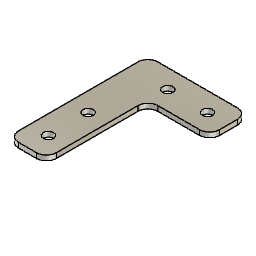
Master v16 (Autodesk Fusion 360 archive; units mm, degrees)
design "Funky Bracket"
Autodesk Fusion 360 part; units mm, degrees
note: some values were not read from the file. Chosen so that the rebuilt part matches the saved one: which face or edge a step refers to. Set by a fixed rule: which sketch regions a step uses.
sketch "Sketch1" plane through (0, 0, 0) normal (0, 0, 1) x (1, 0, 0)
  circle A0 centre (0, -38.1) radius 3.2385
  circle A1 centre (0, -63.5) radius 3.2385
  circle A2 centre (12.7, 0) radius 3.2385
  circle A3 centre (38.1, 0) radius 3.2385
  line L0 (-12.065, 12.065) -> (-12.065, -76.835)
  line L1 (-12.065, -76.835) -> (12.065, -76.835)
  line L2 (12.065, -76.835) -> (12.065, -12.065)
  line L3 (12.065, -12.065) -> (51.435, -12.065)
  line L4 (51.435, -12.065) -> (51.435, 12.065)
  line L5 (51.435, 12.065) -> (-12.065, 12.065)
  line L6 (0, 0) -> (51.435, 0) construction
  line L7 (0, 0) -> (0, -76.835) construction
  dimension "d1" = 6.477
  dimension "d2" = 38.1
  dimension "d4" = 25.4
  dimension "d6" = 12.7
  dimension "d8" = 24.13
  dimension "d9" = 24.13
  dimension "d10" = 88.9
  dimension "d11" = 25.4
  dimension "d12" = 63.5
  constraint equal A0 A1
  constraint equal A0 A2
  constraint equal A2 A3
  constraint vertical L0
  constraint perpendicular L0 L1
  constraint perpendicular L1 L2
  constraint perpendicular L0 L3
  constraint perpendicular L3 L4
  constraint horizontal L5
  constraint coincident L6.start L7.start
  constraint midpoint L4 L6.end
  constraint midpoint L1 L7.end
  constraint vertical L7
  constraint horizontal L6
  measures "d1" diameter of A0
  measures "d2" distance of L6.start A0.centre
  measures "d4" distance of A0.centre A1.centre
  measures "d6" distance of L6.start A2.centre
  measures "d8" distance of L3.end L4.end
  measures "d9" distance of L0.end L1.end
  measures "d10" distance of L0.start L0.end
  measures "d11" distance of A2.centre A3.centre
  measures "d12" distance of L0.start L4.end
extrude "Extrude1" add sketch "Sketch1" along normal blind 3.175
fillet "Fillet1" radius 6.35 6 edges at (12.065, -76.835, 1.5875) (-12.065, -76.835, 1.5875) (-12.065, 12.065, 1.5875) (51.435, -12.065, 1.5875) (51.435, 12.065, 1.5875) (12.065, -12.065, 1.5875)
equation "d13 = ( 1 / 8 ) * 1 in"

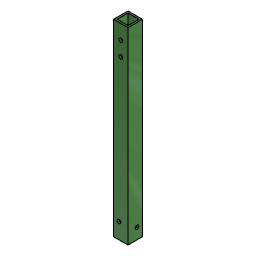
design "Verticle Tube Rear Left"
Autodesk Fusion 360 part; units mm, degrees
imported_body "Derived Base Feature4" makes body 1
imported_body "Derived Base Feature3" makes body 2
sketch "sketch 209" plane through (0, 0, 0) normal (0, 0, 1) x (-1, 0, 0)
  line L0 (-100.8889, 72.7861) -> (-103.3889, 70.7861)
  arc A0 (-109.0111, 77.8139) -> (-103.3889, 70.7861) centre (-106.2, 74.3) ccw
  line L1 (-109.0111, 77.8139) -> (-106.5111, 79.8139)
  arc A1 (-100.8889, 72.7861) -> (-106.5111, 79.8139) centre (-103.7, 76.3) ccw
  line L2 (-106.5111, 821.8861) -> (-109.0111, 823.8861)
  arc A2 (-103.3889, 830.9139) -> (-109.0111, 823.8861) centre (-106.2, 827.4) ccw
  line L3 (-103.3889, 830.9139) -> (-100.8889, 828.9139)
  arc A3 (-106.5111, 821.8861) -> (-100.8889, 828.9139) centre (-103.7, 825.4) ccw
  line L4 (-665.3111, 821.8861) -> (-667.8111, 823.8861)
  arc A4 (-662.1889, 830.9139) -> (-667.8111, 823.8861) centre (-665, 827.4) ccw
  line L5 (-662.1889, 830.9139) -> (-659.6889, 828.9139)
  arc A5 (-665.3111, 821.8861) -> (-659.6889, 828.9139) centre (-662.5, 825.4) ccw
  line L6 (-604.6889, 79.8139) -> (-602.1889, 77.8139)
  arc A6 (-607.8111, 70.7861) -> (-602.1889, 77.8139) centre (-605, 74.3) ccw
  line L7 (-607.8111, 70.7861) -> (-610.3111, 72.7861)
  arc A7 (-604.6889, 79.8139) -> (-610.3111, 72.7861) centre (-607.5, 76.3) ccw
  line L8 (-659.6889, 72.7861) -> (-662.1889, 70.7861)
  arc A8 (-667.8111, 77.8139) -> (-662.1889, 70.7861) centre (-665, 74.3) ccw
  line L9 (-667.8111, 77.8139) -> (-665.3111, 79.8139)
  arc A9 (-659.6889, 72.7861) -> (-665.3111, 79.8139) centre (-662.5, 76.3) ccw
  line L10 (-604.6889, 752.9139) -> (-602.1889, 750.9139)
  arc A10 (-607.8111, 743.8861) -> (-602.1889, 750.9139) centre (-605, 747.4) ccw
  line L11 (-607.8111, 743.8861) -> (-610.3111, 745.8861)
  arc A11 (-604.6889, 752.9139) -> (-610.3111, 745.8861) centre (-607.5, 749.4) ccw
  line L12 (-100.8889, 745.8861) -> (-103.3889, 743.8861)
  arc A12 (-109.0111, 750.9139) -> (-103.3889, 743.8861) centre (-106.2, 747.4) ccw
  line L13 (-109.0111, 750.9139) -> (-106.5111, 752.9139)
  arc A13 (-100.8889, 745.8861) -> (-106.5111, 752.9139) centre (-103.7, 749.4) ccw
  line L14 (-45.8889, 79.8139) -> (-43.3889, 77.8139)
  arc A14 (-49.0111, 70.7861) -> (-43.3889, 77.8139) centre (-46.2, 74.3) ccw
  line L15 (-49.0111, 70.7861) -> (-51.5111, 72.7861)
  arc A15 (-45.8889, 79.8139) -> (-51.5111, 72.7861) centre (-48.7, 76.3) ccw
  line L16 (-106.5111, 148.7861) -> (-109.0111, 150.7861)
  arc A16 (-103.3889, 157.8139) -> (-109.0111, 150.7861) centre (-106.2, 154.3) ccw
  line L17 (-103.3889, 157.8139) -> (-100.8889, 155.8139)
  arc A17 (-106.5111, 148.7861) -> (-100.8889, 155.8139) centre (-103.7, 152.3) ccw
  line L18 (-43.3889, 823.8861) -> (-45.8889, 821.8861)
  arc A18 (-51.5111, 828.9139) -> (-45.8889, 821.8861) centre (-48.7, 825.4) ccw
  line L19 (-51.5111, 828.9139) -> (-49.0111, 830.9139)
  arc A19 (-43.3889, 823.8861) -> (-49.0111, 830.9139) centre (-46.2, 827.4) ccw
  line L20 (-602.1889, 823.8861) -> (-604.6889, 821.8861)
  arc A20 (-610.3111, 828.9139) -> (-604.6889, 821.8861) centre (-607.5, 825.4) ccw
  line L21 (-610.3111, 828.9139) -> (-607.8111, 830.9139)
  arc A21 (-602.1889, 823.8861) -> (-607.8111, 830.9139) centre (-605, 827.4) ccw
  line L22 (-602.1889, 150.7861) -> (-604.6889, 148.7861)
  arc A22 (-610.3111, 155.8139) -> (-604.6889, 148.7861) centre (-607.5, 152.3) ccw
  line L23 (-610.3111, 155.8139) -> (-607.8111, 157.8139)
  arc A23 (-602.1889, 150.7861) -> (-607.8111, 157.8139) centre (-605, 154.3) ccw
  line L24 (-665.3111, 148.7861) -> (-667.8111, 150.7861)
  arc A24 (-662.1889, 157.8139) -> (-667.8111, 150.7861) centre (-665, 154.3) ccw
  line L25 (-662.1889, 157.8139) -> (-659.6889, 155.8139)
  arc A25 (-665.3111, 148.7861) -> (-659.6889, 155.8139) centre (-662.5, 152.3) ccw
  line L26 (-659.6889, 745.8861) -> (-662.1889, 743.8861)
  arc A26 (-667.8111, 750.9139) -> (-662.1889, 743.8861) centre (-665, 747.4) ccw
  line L27 (-667.8111, 750.9139) -> (-665.3111, 752.9139)
  arc A27 (-659.6889, 745.8861) -> (-665.3111, 752.9139) centre (-662.5, 749.4) ccw
  line L28 (-45.8889, 752.9139) -> (-43.3889, 750.9139)
  arc A28 (-49.0111, 743.8861) -> (-43.3889, 750.9139) centre (-46.2, 747.4) ccw
  line L29 (-49.0111, 743.8861) -> (-51.5111, 745.8861)
  arc A29 (-45.8889, 752.9139) -> (-51.5111, 745.8861) centre (-48.7, 749.4) ccw
  line L30 (-43.3889, 150.7861) -> (-45.8889, 148.7861)
  arc A30 (-51.5111, 155.8139) -> (-45.8889, 148.7861) centre (-48.7, 152.3) ccw
  line L31 (-51.5111, 155.8139) -> (-49.0111, 157.8139)
  arc A31 (-43.3889, 150.7861) -> (-49.0111, 157.8139) centre (-46.2, 154.3) ccw
  line L32 (0, 0) -> (0, 889)
  line L33 (0, 889) -> (-711.2, 889)
  line L34 (-711.2, 889) -> (-711.2, 0)
  line L35 (-711.2, 0) -> (0, 0)
  line L36 (0, 25.4) -> (-711.2, 25.4)
  line L37 (-25.4, 0) -> (-25.4, 889)
  line L38 (-685.8, 0) -> (-685.8, 889)
  line L39 (0, 444.5) -> (-25.4, 444.5) construction
  line L40 (-685.8, 444.5) -> (-711.2, 444.5) construction
  line L41 (-355.6, 863.6) -> (-355.6, 889) construction
  line L42 (-25.4, 672.846) -> (-685.8, 672.846) construction
  line L43 (-711.2, 889) -> (0, 889) construction
  line L44 (0, 863.6) -> (-711.2, 863.6) construction
  line L45 (-25.4, 647.446) -> (-685.8, 647.446) construction
  line L46 (-355.6, 672.846) -> (-355.6, 647.446) construction
  line L47 (-355.6, 863.6) -> (-355.6, 672.846) construction
  line L48 (-355.6, 768.223) -> (-304.8, 768.223) construction
  line L49 (-355.6, 768.223) -> (-406.4, 768.223) construction
  line L50 (-25.4, 556.006) -> (-216.154, 556.006) construction
  line L51 (-120.777, 556.006) -> (-120.777, 647.446) construction
  line L52 (-355.6, 25.4) -> (-355.6, 0) construction
  line L53 (-25.4, 672.846) -> (-50.8, 672.846)
  line L54 (-50.8, 672.846) -> (-50.8, 723.646)
  line L55 (-50.8, 723.646) -> (-25.4, 723.646)
  line L56 (-25.4, 723.646) -> (-25.4, 672.846)
  line L57 (-25.4, 698.246) -> (-50.8, 698.246) construction
  line L58 (-25.4, 25.4) -> (-50.8, 25.4)
  line L59 (-50.8, 25.4) -> (-50.8, 50.8)
  line L60 (-50.8, 50.8) -> (-25.4, 50.8)
  line L61 (-25.4, 50.8) -> (-25.4, 25.4)
  line L62 (-25.4, 38.1) -> (-50.8, 38.1) construction
  line L63 (-25.4, 838.2) -> (-50.8, 838.2)
  line L64 (-50.8, 838.2) -> (-50.8, 863.6)
  line L65 (-50.8, 863.6) -> (-25.4, 863.6)
  line L66 (-25.4, 863.6) -> (-25.4, 838.2)
  line L67 (-38.1, 838.2) -> (-38.1, 863.6) construction
extrude "Extrude1" add sketch "sketch 209" along normal blind 330.2 separate body contours L36 L37 L58 L59 L60 L61 makes body 3
shell "Shell1" thickness 3.175 removed faces 1 at (42.3333, -42.3333, 330.2) on bodies 3
extrude "Extrude2" cut 1 faces at (34.925, -34.925, 3.175) along direction (0, 0, -1) blind 21.0058 on bodies 3 bodies 3
sketch "Sketch1" plane through (50.8, 0, 0) normal (1, 0, 0) x (0, 1, 0)
  line L0 (-50.8, 0) -> (-25.4, 0)
  line L1 (-25.4, 0) -> (-25.4, 330.2)
  line L2 (-25.4, 330.2) -> (-50.8, 330.2)
  line L3 (-50.8, 330.2) -> (-50.8, 0)
  circle A0 centre (-34.925, 19.05) radius 3.302
extrude "Extrude3" cut sketch "Sketch1" against normal blind 179.324 contours A0 bodies 3
sketch "Sketch2" plane through (0, -50.8, 0) normal (0, -1, 0) x (1, 0, 0)
  line L0 (25.4, 0) -> (50.8, 0)
  line L1 (50.8, 0) -> (50.8, 330.2)
  line L2 (50.8, 330.2) -> (25.4, 330.2)
  line L3 (25.4, 330.2) -> (25.4, 0)
  circle A0 centre (38.1, 304.8) radius 3.2385
  circle A1 centre (38.1, 279.4) radius 3.2385
extrude "Extrude4" cut sketch "Sketch2" against normal blind 66.7512 contours A0 | A1 bodies 3
sketch "Sketch3" plane through (0, -25.4, 0) normal (0, 1, 0) x (-1, 0, 0)
  circle A0 centre (-38.1, 304.8) radius 3.2385
  circle A1 centre (-38.1, 279.4) radius 3.2385
  line L0 (-50.8, 0) -> (-25.4, 0)
  line L1 (-25.4, 0) -> (-25.4, 330.2)
  line L2 (-25.4, 330.2) -> (-50.8, 330.2)
  line L3 (-50.8, 330.2) -> (-50.8, 0)
  circle A2 centre (-41.275, 27.94) radius 3.302
  line L4 (-38.1, 0) -> (-38.1, 35.56) construction
  circle A3 centre (-34.925, 27.94) radius 3.302
  constraint midpoint L0 L4.start
  constraint perpendicular L0 L4
  constraint symmetric A2 L4 A3
extrude "Extrude5" cut sketch "Sketch3" against normal blind 194.056 contours A2 A3 | A2 A3 picked at (-38.1364, 28.1946) picked at (-33.7509, 28.097) bodies 3
hidden bodies 2 1
equation "floorToTray = 13 in"
equation "d2 = floorToTray"
named bodies: "Body1 (Context3)", "Body1 (Context4)"
